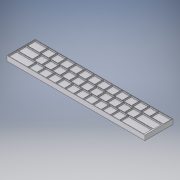
# Autodesk Inventor part: keyboard-base_standard
Saved by Autodesk Inventor 2016 (Build 200138000, 138)
## iProperties
Created: 2016-12-08
Part Number: keyboard-base_standard
Material: Generic
Document SubType Name: Modeling
Designer: Cemra JC
Density: 1 g/cm^3
Appearance: Default
Author: Cemra JC
Autodesk Inventor part; units mm, degrees
ref_plane "YZ Plane" through (0, 0, 0) normal (1, 0, 0) x (0, 1, 0)
ref_plane "XZ Plane" through (0, 0, 0) normal (0, 1, 0) x (-1, 0, 0)
ref_plane "XY Plane" through (0, 0, 0) normal (0, 0, 1) x (1, 0, 0)
sketch "Keyboard Backplane" plane through (0, 0, 0) normal (0, 1, 0) x (-1, 0, 0)
  line L0 (143.25, 29.175) -> (-143.25, 29.175)
  line L1 (-143.25, 29.175) -> (-143.25, -29.175)
  line L2 (-143.25, -29.175) -> (143.25, -29.175)
  line L3 (143.25, -29.175) -> (143.25, 29.175)
  line L4 (143.25, 29.175) -> (-143.25, -29.175) construction
  line L5 (-143.25, 29.175) -> (143.25, -29.175) construction
  point P0 (0, 0)
  point P1 (0, 0)
  dimension "d0" = 58.35
  dimension "d1" = 286.5
  constraints: 12 end point, 2 parallel, 1 coincident, 1 horizontal, 1 midpoint, 1 perpendicular
  measures "d0" distance of L0.end L1.end
  measures "d1" distance of L1.end L2.end
extrude "Keyboard Backplane Body" add sketch "Keyboard Backplane" along normal blind 10
sketch "KeyCap Outlines" plane through (0, 10, 0) normal (0, 1, 0) x (1, 0, 0)
  line L0 (-142.25, 28.175) -> (-115.1, 28.175)
  line L1 (-115.1, 28.175) -> (-115.1, 10.075)
  line L2 (-115.1, 10.075) -> (-142.25, 10.075)
  line L3 (-142.25, 10.075) -> (-142.25, 28.175)
  line L4 (-143.25, -29.175) -> (143.25, -29.175) projected
  line L5 (143.25, -29.175) -> (143.25, 29.175) projected
  line L6 (143.25, 29.175) -> (-143.25, 29.175) projected
  line L7 (-143.25, 29.175) -> (-143.25, -29.175) projected
  line L8 (-114.1, 10.075) -> (-96, 10.075)
  line L9 (-96, 10.075) -> (-96, 28.175)
  line L10 (-96, 28.175) -> (-114.1, 28.175)
  line L11 (-114.1, 28.175) -> (-114.1, 10.075)
  line L12 (-95, 10.075) -> (-76.9, 10.075)
  line L13 (-76.9, 10.075) -> (-76.9, 28.175)
  line L14 (-76.9, 28.175) -> (-95, 28.175)
  line L15 (-95, 28.175) -> (-95, 10.075)
  line L16 (-75.9, 10.075) -> (-57.8, 10.075)
  line L17 (-57.8, 10.075) -> (-57.8, 28.175)
  line L18 (-57.8, 28.175) -> (-75.9, 28.175)
  line L19 (-75.9, 28.175) -> (-75.9, 10.075)
  line L20 (-56.8, 10.075) -> (-38.7, 10.075)
  line L21 (-38.7, 10.075) -> (-38.7, 28.175)
  line L22 (-38.7, 28.175) -> (-56.8, 28.175)
  line L23 (-56.8, 28.175) -> (-56.8, 10.075)
  line L24 (-37.7, 10.075) -> (-19.6, 10.075)
  line L25 (-19.6, 10.075) -> (-19.6, 28.175)
  line L26 (-19.6, 28.175) -> (-37.7, 28.175)
  line L27 (-37.7, 28.175) -> (-37.7, 10.075)
  line L28 (-18.6, 10.075) -> (-0.5, 10.075)
  line L29 (-0.5, 10.075) -> (-0.5, 28.175)
  line L30 (-0.5, 28.175) -> (-18.6, 28.175)
  line L31 (-18.6, 28.175) -> (-18.6, 10.075)
  line L32 (0.5, 10.075) -> (18.6, 10.075)
  line L33 (18.6, 10.075) -> (18.6, 28.175)
  line L34 (18.6, 28.175) -> (0.5, 28.175)
  line L35 (0.5, 28.175) -> (0.5, 10.075)
  line L36 (19.6, 10.075) -> (37.7, 10.075)
  line L37 (37.7, 10.075) -> (37.7, 28.175)
  line L38 (37.7, 28.175) -> (19.6, 28.175)
  line L39 (19.6, 28.175) -> (19.6, 10.075)
  line L40 (38.7, 10.075) -> (56.8, 10.075)
  line L41 (56.8, 10.075) -> (56.8, 28.175)
  line L42 (56.8, 28.175) -> (38.7, 28.175)
  line L43 (38.7, 28.175) -> (38.7, 10.075)
  line L44 (57.8, 10.075) -> (75.9, 10.075)
  line L45 (75.9, 10.075) -> (75.9, 28.175)
  line L46 (75.9, 28.175) -> (57.8, 28.175)
  line L47 (57.8, 28.175) -> (57.8, 10.075)
  line L48 (76.9, 10.075) -> (95, 10.075)
  line L49 (95, 10.075) -> (95, 28.175)
  line L50 (95, 28.175) -> (76.9, 28.175)
  line L51 (76.9, 28.175) -> (76.9, 10.075)
  line L52 (96, 10.075) -> (114.1, 10.075)
  line L53 (114.1, 10.075) -> (114.1, 28.175)
  line L54 (114.1, 28.175) -> (96, 28.175)
  line L55 (96, 28.175) -> (96, 10.075)
  line L56 (115.1, 28.175) -> (142.25, 28.175)
  line L57 (142.25, 28.175) -> (142.25, 10.075)
  line L58 (142.25, 10.075) -> (115.1, 10.075)
  line L59 (115.1, 10.075) -> (115.1, 28.175)
  line L60 (-142.25, 9.075) -> (-110.57, 9.075)
  line L61 (-110.57, 9.075) -> (-110.57, -9.025)
  line L62 (-110.57, -9.025) -> (-142.25, -9.025)
  line L63 (-142.25, -9.025) -> (-142.25, 9.075)
  line L64 (-109.57, -9.025) -> (-91.47, -9.025)
  line L65 (-91.47, -9.025) -> (-91.47, 9.075)
  line L66 (-91.47, 9.075) -> (-109.57, 9.075)
  line L67 (-109.57, 9.075) -> (-109.57, -9.025)
  line L68 (-72.37, -9.025) -> (-72.37, 9.075)
  line L69 (-72.37, 9.075) -> (-90.47, 9.075)
  line L70 (-90.47, 9.075) -> (-90.47, -9.025)
  line L71 (-90.47, -9.025) -> (-72.37, -9.025)
  line L72 (-53.27, -9.025) -> (-53.27, 9.075)
  line L73 (-53.27, 9.075) -> (-71.37, 9.075)
  line L74 (-71.37, 9.075) -> (-71.37, -9.025)
  line L75 (-71.37, -9.025) -> (-53.27, -9.025)
  line L76 (-34.17, -9.025) -> (-34.17, 9.075)
  line L77 (-34.17, 9.075) -> (-52.27, 9.075)
  line L78 (-52.27, 9.075) -> (-52.27, -9.025)
  line L79 (-52.27, -9.025) -> (-34.17, -9.025)
  line L80 (-15.07, -9.025) -> (-15.07, 9.075)
  line L81 (-15.07, 9.075) -> (-33.17, 9.075)
  line L82 (-33.17, 9.075) -> (-33.17, -9.025)
  line L83 (-33.17, -9.025) -> (-15.07, -9.025)
  line L84 (4.03, -9.025) -> (4.03, 9.075)
  line L85 (4.03, 9.075) -> (-14.07, 9.075)
  line L86 (-14.07, 9.075) -> (-14.07, -9.025)
  line L87 (-14.07, -9.025) -> (4.03, -9.025)
  line L88 (23.13, -9.025) -> (23.13, 9.075)
  line L89 (23.13, 9.075) -> (5.03, 9.075)
  line L90 (5.03, 9.075) -> (5.03, -9.025)
  line L91 (5.03, -9.025) -> (23.13, -9.025)
  line L92 (42.23, -9.025) -> (42.23, 9.075)
  line L93 (42.23, 9.075) -> (24.13, 9.075)
  line L94 (24.13, 9.075) -> (24.13, -9.025)
  line L95 (24.13, -9.025) -> (42.23, -9.025)
  line L96 (61.33, -9.025) -> (61.33, 9.075)
  line L97 (61.33, 9.075) -> (43.23, 9.075)
  line L98 (43.23, 9.075) -> (43.23, -9.025)
  line L99 (43.23, -9.025) -> (61.33, -9.025)
  line L100 (80.43, -9.025) -> (80.43, 9.075)
  line L101 (80.43, 9.075) -> (62.33, 9.075)
  line L102 (62.33, 9.075) -> (62.33, -9.025)
  line L103 (62.33, -9.025) -> (80.43, -9.025)
  line L104 (99.53, -9.025) -> (99.53, 9.075)
  line L105 (99.53, 9.075) -> (81.43, 9.075)
  line L106 (81.43, 9.075) -> (81.43, -9.025)
  line L107 (81.43, -9.025) -> (99.53, -9.025)
  line L108 (100.53, 9.075) -> (141.26, 9.075)
  line L109 (141.26, 9.075) -> (141.26, -9.025)
  line L110 (141.26, -9.025) -> (100.53, -9.025)
  line L111 (100.53, -9.025) -> (100.53, 9.075)
  line L112 (-142.25, -10.025) -> (-101.52, -10.025)
  line L113 (-101.52, -10.025) -> (-101.52, -28.125)
  line L114 (-101.52, -28.125) -> (-142.25, -28.125)
  line L115 (-142.25, -28.125) -> (-142.25, -10.025)
  line L116 (-100.52, -10.025) -> (-82.42, -10.025)
  line L117 (-82.42, -10.025) -> (-82.42, -28.125)
  line L118 (-82.42, -28.125) -> (-100.52, -28.125)
  line L119 (-100.52, -28.125) -> (-100.52, -10.025)
  line L120 (-63.32, -28.125) -> (-81.42, -28.125)
  line L121 (-63.32, -10.025) -> (-63.32, -28.125)
  line L122 (-81.42, -28.125) -> (-81.42, -10.025)
  line L123 (-81.42, -10.025) -> (-63.32, -10.025)
  line L124 (-44.22, -28.125) -> (-62.32, -28.125)
  line L125 (-44.22, -10.025) -> (-44.22, -28.125)
  line L126 (-62.32, -28.125) -> (-62.32, -10.025)
  line L127 (-62.32, -10.025) -> (-44.22, -10.025)
  line L128 (-25.12, -28.125) -> (-43.22, -28.125)
  line L129 (-25.12, -10.025) -> (-25.12, -28.125)
  line L130 (-43.22, -28.125) -> (-43.22, -10.025)
  line L131 (-43.22, -10.025) -> (-25.12, -10.025)
  line L132 (-6.02, -28.125) -> (-24.12, -28.125)
  line L133 (-6.02, -10.025) -> (-6.02, -28.125)
  line L134 (-24.12, -28.125) -> (-24.12, -10.025)
  line L135 (-24.12, -10.025) -> (-6.02, -10.025)
  line L136 (13.08, -28.125) -> (-5.02, -28.125)
  line L137 (13.08, -10.025) -> (13.08, -28.125)
  line L138 (-5.02, -28.125) -> (-5.02, -10.025)
  line L139 (-5.02, -10.025) -> (13.08, -10.025)
  line L140 (32.18, -28.125) -> (14.08, -28.125)
  line L141 (32.18, -10.025) -> (32.18, -28.125)
  line L142 (14.08, -28.125) -> (14.08, -10.025)
  line L143 (14.08, -10.025) -> (32.18, -10.025)
  line L144 (51.28, -28.125) -> (33.18, -28.125)
  line L145 (51.28, -10.025) -> (51.28, -28.125)
  line L146 (33.18, -28.125) -> (33.18, -10.025)
  line L147 (33.18, -10.025) -> (51.28, -10.025)
  line L148 (70.38, -28.125) -> (52.28, -28.125)
  line L149 (70.38, -10.025) -> (70.38, -28.125)
  line L150 (52.28, -28.125) -> (52.28, -10.025)
  line L151 (52.28, -10.025) -> (70.38, -10.025)
  line L152 (89.48, -28.125) -> (71.38, -28.125)
  line L153 (89.48, -10.025) -> (89.48, -28.125)
  line L154 (71.38, -28.125) -> (71.38, -10.025)
  line L155 (71.38, -10.025) -> (89.48, -10.025)
  line L156 (90.48, -28.125) -> (139.96, -28.125)
  line L157 (139.96, -28.125) -> (139.96, -10.025)
  line L158 (139.96, -10.025) -> (90.48, -10.025)
  line L159 (90.48, -10.025) -> (90.48, -28.125)
  point P0 (0, 0)
  dimension "d4" = 27.15
  dimension "d5" = 18.1
  dimension "d6" = 1
  dimension "d7" = 1
  dimension "d8" = 18.1
  dimension "d9" = 18.1
  dimension "d10" = 1
  dimension "d11" = 1
  dimension "d14" = 19.1
  dimension "d19" = 27.15
  dimension "d20" = 18.1
  dimension "d21" = 1
  dimension "d22" = 1
  dimension "d23" = 18.1
  dimension "d24" = 31.68
  dimension "d25" = 1
  dimension "d26" = 1
  dimension "d27" = 18.1
  dimension "d28" = 18.1
  dimension "d29" = 1
  dimension "d30" = 1
  dimension "d33" = 19.1
  dimension "d38" = 18.1
  dimension "d39" = 40.73
  dimension "d40" = 1
  dimension "d41" = 1
  dimension "d42" = 18.1
  dimension "d43" = 40.73
  dimension "d44" = 1
  dimension "d45" = 1
  dimension "d46" = 18.1
  dimension "d47" = 18.1
  dimension "d48" = 1
  dimension "d49" = 1
  dimension "d52" = 19.1
  dimension "d57" = 18.1
  dimension "d58" = 49.48
  dimension "d59" = 1
  dimension "d60" = 1
  constraints: 312 end point, 18 parallel, 12 horizontal, 9 perpendicular, 3 collinear, 237 other
  measures "d4" distance of L1.end L2.end
  measures "d5" distance of L0.end L1.end
  measures "d6" distance between parallel lines of L6 L0
  measures "d7" distance between parallel lines of L7 L3
  measures "d8" distance of L10.end L9.end
  measures "d9" distance of L9.end L8.end
  measures "d10" distance between parallel lines of L6 L10
  measures "d11" distance between parallel lines of L1 L11
  measures "d14" distance of L8.start L12.start
  measures "d19" distance of L57.end L58.end
  measures "d20" distance of L56.end L57.end
  measures "d21" distance between parallel lines of L6 L56
  measures "d22" distance between parallel lines of L53 L59
  measures "d23" distance of L60.end L61.end
  measures "d24" distance of L61.end L62.end
  measures "d25" distance between parallel lines of L2 L60
  measures "d26" distance between parallel lines of L7 L63
  measures "d27" distance of L65.end L66.end
  measures "d28" distance of L64.end L65.end
  measures "d29" distance between parallel lines of L8 L66
  measures "d30" distance between parallel lines of L61 L67
  measures "d33" distance of L64.end L68.start
  measures "d38" distance of L108.end L109.end
  measures "d39" distance of L109.end L110.end
  measures "d40" distance between parallel lines of L104 L111
  measures "d41" distance between parallel lines of L58 L108
  measures "d42" distance of L112.end L113.end
  measures "d43" distance of L113.end L114.end
  measures "d44" distance between parallel lines of L7 L115
  measures "d45" distance between parallel lines of L62 L112
  measures "d46" distance of L116.end L117.end
  measures "d47" distance of L117.end L118.end
  measures "d48" distance between parallel lines of L113 L119
  measures "d49" distance between parallel lines of L64 L116
  measures "d52" distance of L117.end L120.start
  measures "d57" distance of L156.end L157.end
  measures "d58" distance of L156.start L156.end
  measures "d59" distance between parallel lines of L153 L159
  measures "d60" distance between parallel lines of L110 L158
extrude "Keycap Holes" cut sketch "KeyCap Outlines" against normal blind 3 contours L0 L1 L2 L3 | L11 L10 L9 L8 | L15 L14 L13 L12 | L19 L18 L17 L16 | L23 L22 L21 L20 | L27 L26 L25 L24 | L31 L30 L29 L28 | L35 L34 L33 L32 | L39 L38 L37 L36 | L43 L42 L41 L40 | L47 L46 L45 L44 | L51 L50 L49 L48 | L55 L54 L53 L52 | L56 L57 L58 L59 | L60 L61 L62 L63 | L67 L66 L65 L64 | L71 L70 L69 L68 | L75 L74 L73 L72 | L79 L78 L77 L76 | L83 L82 L81 L80 | L87 L86 L85 L84 | L91 L90 L89 L88 | L95 L94 L93 L92 | L99 L98 L97 L96 | L103 L102 L101 L100 | L107 L106 L105 L104 | L108 L109 L110 L111 | L112 L113 L114 L115 | L116 L117 L118 L119 | L120 L122 L123 L121 | L124 L126 L127 L125 | L128 L130 L131 L129 | L132 L134 L135 L133 | L136 L138 L139 L137 | L140 L142 L143 L141 | L144 L146 L147 L145 | L148 L150 L151 L149 | L152 L154 L155 L153 | L159 L158 L157 L156
equation "\"d6\" = d7"
equation "\"d8\" = d5"
equation "\"d9\" = d5"
equation "\"d10\" = d6"
equation "\"d11\" = d7"
equation "\"d19\" = d4"
equation "\"d21\" = d7"
equation "\"d22\" = d7"
equation "\"d23\" = d5"
equation "\"d25\" = d7"
equation "\"d26\" = d7"
equation "\"d27\" = d5"
equation "\"d28\" = d5"
equation "\"d33\" = d27 + d7"
equation "\"d38\" = d5"
equation "\"d40\" = d7"
equation "\"d41\" = d7"
equation "\"d42\" = d5"
equation "\"d43\" = d39"
equation "\"d44\" = d7"
equation "\"d45\" = d7"
equation "\"d46\" = d5"
equation "\"d47\" = d5"
equation "\"d48\" = d7"
equation "\"d49\" = d7"
equation "\"d52\" = d47 + d48"
equation "\"d57\" = d5"
equation "\"d59\" = d7"
equation "\"d60\" = d7"
body "Solid1"
